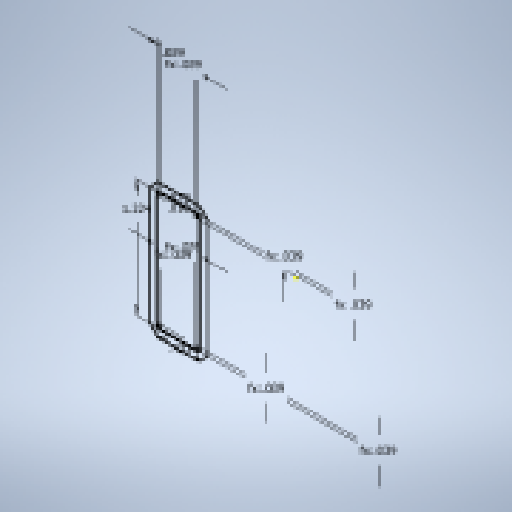
# Autodesk Inventor part: CattailShellMockup_01
Saved by Autodesk Inventor 2024 (Build 280153000, 153)
## iProperties
Created: 2023-12-02
Part Number: CattailShellMockup_01
Material: Generic
Document SubType Name: Modeling
Designer: jevan
Density: 1 g/cm^3
Appearance: Default
Author: jevan
Autodesk Inventor part; units mm, degrees
ref_plane "YZ Plane" through (0, 0, 0) normal (1, 0, 0) x (0, 1, 0)
ref_plane "XZ Plane" through (0, 0, 0) normal (0, 1, 0) x (-1, 0, 0)
ref_plane "XY Plane" through (0, 0, 0) normal (0, 0, 1) x (1, 0, 0)
sketch "Sketch1" plane through (0, 0, 0) normal (0, 0, 1) x (1, 0, 0)
  line L0 (-35.5556, 1.5189) -> (-26.5556, 1.5189)
  line L1 (-25.5556, 0.5189) -> (-25.5556, -28.5811)
  line L2 (-26.5556, -29.5811) -> (-35.5556, -29.5811)
  line L3 (-36.5556, -28.5811) -> (-36.5556, 0.5189)
  line L4 (-35.5556, 1.5189) -> (-36.5556, 0.5189)
  line L5 (-25.5556, 0.5189) -> (-26.5556, 1.5189)
  line L6 (-25.5556, -28.5811) -> (-26.5556, -29.5811)
  line L7 (-35.5556, -29.5811) -> (-36.5556, -28.5811)
  line L8 (-26.452, 1.7689) -> (-25.3056, 0.6224)
  line L9 (-25.3056, 0.6224) -> (-25.3056, -28.6847)
  line L10 (-25.3056, -28.6847) -> (-26.452, -29.8311)
  line L11 (-26.452, -29.8311) -> (-35.6592, -29.8311)
  line L12 (-35.6592, -29.8311) -> (-36.8056, -28.6847)
  line L13 (-36.8056, -28.6847) -> (-36.8056, 0.6224)
  line L14 (-36.8056, 0.6224) -> (-35.6592, 1.7689)
  line L15 (-35.6592, 1.7689) -> (-26.452, 1.7689)
  line L16 (-25.6236, 3.7689) -> (-23.3056, 1.4508)
  line L17 (-23.3056, 1.4508) -> (-23.3056, -29.5131)
  line L18 (-23.3056, -29.5131) -> (-25.6236, -31.8311)
  line L19 (-25.6236, -31.8311) -> (-36.4876, -31.8311)
  line L20 (-36.4876, -31.8311) -> (-38.8056, -29.5131)
  line L21 (-38.8056, -29.5131) -> (-38.8056, 1.4508)
  line L22 (-38.8056, 1.4508) -> (-36.4876, 3.7689)
  line L23 (-36.4876, 3.7689) -> (-25.6236, 3.7689)
  point P0 (0, 0)
  point P1 (-36.5556, 1.5189)
  point P2 (-25.5556, -29.5811)
  point P3 (-25.5556, 1.5189)
  point P4 (-36.5556, -29.5811)
  dimension "d0" = 31.1
  dimension "d1" = 11
  dimension "d2" = 1
  dimension "d3" = 1
  dimension "d4" = 1
  dimension "d5" = 1
  dimension "d6" = 1
  dimension "d7" = 1
  dimension "d8" = 1
  dimension "d9" = 1
  dimension "d10" = 0.25
  dimension "d11" = 2
  constraints: 48 end point, 8 point on line, 6 parallel, 3 perpendicular, 1 horizontal, 15 other
  measures "d0" distance of point (-36.556, -29.581) point (-36.556, 1.519)
  measures "d1" distance of point (-25.556, -29.581) point (-36.556, -29.581)
  measures "d2" distance of L0.start point (-36.556, 1.519)
  measures "d3" distance of L3.end point (-36.556, 1.519)
  measures "d4" distance of L1.start point (-25.556, 1.519)
  measures "d5" distance of L0.end point (-25.556, 1.519)
  measures "d6" distance of L1.end point (-25.556, -29.581)
  measures "d7" distance of L2.start point (-25.556, -29.581)
  measures "d8" distance of L2.end point (-36.556, -29.581)
  measures "d9" distance of L3.start point (-36.556, -29.581)
  measures "d10" distance between parallel lines of L0 L15
  measures "d11" distance between parallel lines of L15 L23
extrude "Extrusion1" add sketch "Sketch1" along normal blind 1.5 contours L0 L5 L1 L6 L2 L7 L3 L4 | L8 L9 L10 L11 L12 L13 L14 L15 | L16 L17 L18 L19 L20 L21 L22 L23
extrude "Extrusion2" add sketch "Sketch1" against normal blind 8 contours L16 L17 L18 L19 L20 L21 L22 L23
equation "\"d3\" = d2"
equation "\"d4\" = d2"
equation "\"d5\" = d4"
equation "\"d6\" = d2"
equation "\"d7\" = d6"
equation "\"d8\" = d2"
equation "\"d9\" = d8"
body "Solid1"
